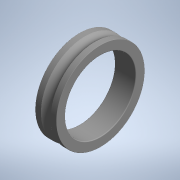
# Autodesk Inventor part: 16006_PART1
Saved by Autodesk Inventor 2020 (Build 240168000, 168)
## iProperties
Part Number: 16006_PART1
Material: Generic
Catalog Web Link: www.cadenas.de
Description: -Deep groove ball bearings
Vendor: SKF
Document SubType Name: Modeling
Designer: partserver
Manufacturer: SKF
Mass: 3.42363 g
Surface Area: 27.2849 cm^2
Volume: 3.42363 cm^3
Density: 1 g/cm^3
Appearance: PSOLRGB-175-175-175
Category: PARTsolutions
Company: SKF
PSOL_IDENT_0: {$CADENAS_DATA\23d-libs\skf\bearings_units_and_housings\ball_bearings\deep_groove_ball_bearings\bb1_
PSOL_IDENT_1: 001_101.prj},188 {VTYP=3D},{NB=16006_PART1},{LINA=16006_PART1},{NN=BB1_001_101_PART1},{NOPRJ=TRUE},{
PSOL_IDENT_2: DATE=10.08.2020 12:45:09},{GEOMDATE=17.06.2020 07:40:43},{VERSION=},{LINEID=4390},{WBVAR=},{WBNUMERI
PSOL_IDENT_3: C=}  {NB=16006_PART1},{LINA=16006_PART1},{KT=DUMMY},{DESIGNATION=16006},{DD=30.000},{D=55.000},{B=9.
PSOL_IDENT_4: 000},{C=0.000},{DD1=37.70},{DD2=0.00},{D1=47.30},{D2=0.00},{D3=0.000},{D4=0.000},{HH=MIN},{BB=0.000}
PSOL_IDENT_5: ,{FF=0.00},{R0MAX=MIN},{R0=MIN},{R12=0.30},{PITCH=42.50},{DW=6.350},{DDAMIN=32.000},{DDAMAX=MIN},{DD
PSOL_IDENT_6: BMIN=MIN},{DDBMAX=MIN},{DBMIN=MIN},{DAMAX=53.000},{BBAMIN=MIN},{CAMAX=MIN},{RAMAX=0.300},{LOAD1=11.9
PSOL_IDENT_7: 00},{LOAD2=7.350},{LOAD3=0.310},{SPEED1=28000},{SPEED2=17000},{KR=0.020},{F0=15.000},{Z=12},{II=1},{
PSOL_IDENT_8: MASS=0.089},{BEARING=16006},{RING=},{HELP=3.850},{HELP2=3.850},{DD1ALG=18.850},{YALG=18.850},{PITCH1=
PSOL_IDENT_9: 42.500},{DW1=6.350},{YALG1=23.650},{HALG1=3.850},{SH=18.850},{CU=0.530},{DESIGN=dgbb1},{HALG=3.85},{
PSOL_IDENT_10: B1=0},{SHIELDHELP=1}
NB: 16006_PART1
NT: Deep groove ball bearings
NBSYN: $DESIGNATION._PART1
LINA: 16006_PART1
CATALOG: SKF
SUPPLIER: SKF
ARTICLENO: 16006_PART1
BOMINFO: 16006_PART1
CREATOR: CADENAS GmbH
Title: 16006_PART1
Author: Cadenas PARTsolutions
Comments: Deep groove ball bearings
Autodesk Inventor part; units mm, degrees
ref_plane "YZ Plane" through (0, 0, 0) normal (1, 0, 0) x (0, 1, 0)
ref_plane "XZ Plane" through (0, 0, 0) normal (0, 1, 0) x (-1, 0, 0)
ref_plane "XY Plane" through (0, 0, 0) normal (0, 0, 1) x (1, 0, 0)
sketch "Sketch_54" plane through (0, 0, 0) normal (0, 0, 1) x (1, 0, 0)
  line L0 (100, 0) -> (-100, 0)
  arc A0 (0, 15.3) -> (0.3, 15) centre (0.3, 15.3) ccw
  line L1 (0.3, 15) -> (8.7, 15)
  arc A1 (8.7, 15) -> (9, 15.3) centre (8.7, 15.3) ccw
  line L2 (9, 15.3) -> (9, 18.75)
  arc A2 (9, 18.75) -> (8.9, 18.85) centre (8.9, 18.75) ccw
  line L3 (8.9, 18.85) -> (6.5786, 18.85)
  arc A3 (2.4214, 18.85) -> (6.5786, 18.85) centre (4.5, 21.25) ccw
  line L4 (2.4214, 18.85) -> (0.1, 18.85)
  arc A4 (0.1, 18.85) -> (0, 18.75) centre (0.1, 18.75) ccw
  line L5 (0, 18.75) -> (0, 15.3)
  constraints: 12 end point, 10 point on circle, 5 centre point
revolve "Revolution1" add sketch "Sketch_54" angle 360 about axis through (100, 0, 0) along (1, 0, 0)
body "Solid1"
